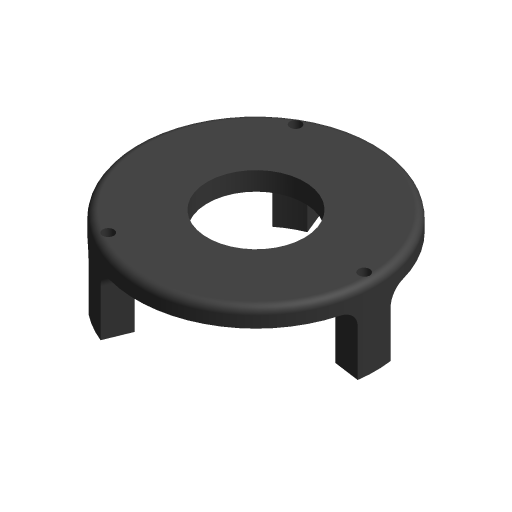
# Autodesk Inventor part: Engine retention
Saved by Autodesk Inventor 2024 (Build 280153000, 153)
## iProperties
Part Number: Engine retention
Material: Generic
Document SubType Name: Modeling
Designer: Jamie
Appearance: Default
Author: Jamie
Autodesk Inventor part; units mm, degrees
ref_plane "YZ Plane" through (0, 0, 0) normal (1, 0, 0) x (0, 1, 0)
ref_plane "XZ Plane" through (0, 0, 0) normal (0, 1, 0) x (-1, 0, 0)
ref_plane "XY Plane" through (0, 0, 0) normal (0, 0, 1) x (1, 0, 0)
sketch "Sketch1" plane through (0, 0, 0) normal (0, 1, 0) x (-1, 0, 0)
  circle A0 centre (0, 0) radius 25
  circle A1 centre (0, 0) radius 32
  dimension "d0" = 50
  dimension "d1" = 64
  constraints: 2 centre point, 2 coincident
  measures "d0" diameter of A0
  measures "d1" diameter of A1
extrude "Extrusion1" add sketch "Sketch1" along normal blind 16.5
sketch "Sketch2" plane through (0, 16.5, 0) normal (0, 1, 0) x (1, 0, 0)
  circle A0 centre (0, 0) radius 13
  circle A1 centre (0, 0) radius 32
  dimension "d4" = 26
  constraints: 2 centre point, 2 coincident
  measures "d4" diameter of A0
extrude "Extrusion2" add sketch "Sketch2" along normal blind 5
sketch "Sketch4" plane through (0, 0, 0) normal (0, -1, 0) x (1, 0, 0)
  circle A0 centre (29, 0) radius 1.5
  circle A1 centre (0, 0) radius 25 projected
  circle A2 centre (0, 0) radius 32 projected
  dimension "d7" = 3
  dimension "d9" = 29
  constraints: 1 centre point
  measures "d7" diameter of A0
  measures "d9" distance of A2.centre A0.centre
extrude "Extrusion3" cut sketch "Sketch4" against normal through all contours A0
pattern_circular "Circular Pattern1" count 3 over 360 about axis through (0, 0, 0) along (0, 1, 0) of "Extrusion3"
sketch "Sketch5" plane through (0, 0, 0) normal (0, -1, 0) x (1, 0, 0)
  line L0 (0, 0) -> (36.6386, -5.1024)
  line L1 (36.6386, -5.1024) -> (37.4304, -25.9892)
  line L2 (37.4304, -25.9892) -> (-15.9101, -39.2371)
  circle A0 centre (0, 0) radius 32 projected
  line L3 (-15.9101, -39.2371) -> (0, 0)
  circle A1 centre (29, 0) radius 1.5 projected
  circle A2 centre (-14.5, -25.1147) radius 1.5 projected
  point P0 (-12.0246, -29.6548)
  point P1 (31.6941, -4.4138)
  dimension "d15" = 4
  dimension "d22" = 4
  constraints: 8 end point
  measures "d15" distance from line of A1.centre L0
  measures "d22" distance from line of A2.centre L3
extrude "Extrusion4" cut sketch "Sketch5" against normal blind 16.5 contours L0 A0 L3 picked at (12.6104, -17.0364)
pattern_circular "Circular Pattern2" count 3 over 360 about axis through (0, 16.5, 0) along (0, 1, 0) of "Extrusion4"
fillet "Fillet1" radius 4 6 edges at (28.2276, 16.5, -3.931) (-10.7094, 16.5, -26.4113) (-17.5182, 16.5, -22.4803) (-17.5182, 16.5, 22.4803) (-10.7094, 16.5, 26.4113) (28.2276, 16.5, 3.931)
fillet "Fillet2" radius 2 1 edges at (32, 21.5, 0)
body "Solid1"
